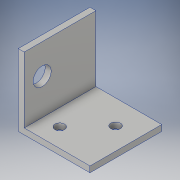
# Autodesk Inventor part: CLB_085_ClimberMountLBracket
Saved by Autodesk Inventor 2018.3 (Build 223284000, 284)
## iProperties
Created: 2020-02-22
Part Number: CLB_085_ClimberMountLBracket
Material: Aluminum 6061
Document SubType Name: Modeling
Designer: 22perngrac
Density: 2.7 g/cm^3
Appearance: Aluminum - Flat
Mass: 22.9264 g
Surface Area: 62.4575 cm^2
Volume: 8.49126 cm^3
Author: 22perngrac
Autodesk Inventor part; units mm, degrees
ref_plane "YZ Plane" through (0, 0, 0) normal (1, 0, 0) x (0, 1, 0)
ref_plane "XZ Plane" through (0, 0, 0) normal (0, 1, 0) x (-1, 0, 0)
ref_plane "XY Plane" through (0, 0, 0) normal (0, 0, 1) x (1, 0, 0)
sketch "Sketch1" plane through (0, 0, 0) normal (0, 0, 1) x (1, 0, 0)
  line L0 (0, 0) -> (0, 38.1)
  line L1 (0, 38.1) -> (3.175, 38.1)
  line L2 (3.175, 38.1) -> (3.175, 3.175)
  line L3 (3.175, 3.175) -> (38.1, 3.175)
  line L4 (38.1, 3.175) -> (38.1, 0)
  line L5 (38.1, 0) -> (0, 0)
  dimension "d0" = 38.1
  dimension "d1" = 3.175
  constraints: 12 end point, 7 perpendicular, 1 vertical
  measures "d0" distance of L4.end L0.start
  measures "d1" distance of L3.end L4.end
extrude "Extrusion1" add sketch "Sketch1" along normal blind 38.1
sketch "Sketch2" plane through (3.175, 3.175, 0) normal (1, 0, 0) x (0, 0, -1)
  line L0 (0, 34.925) -> (-38.1, 34.925) projected
  line L1 (-38.1, 0) -> (-38.1, 34.925) projected
  line L2 (0, 0) -> (-38.1, 0) projected
  point P0 (0, -3.175)
  point P1 (-28.575, 19.05)
  dimension "d5" = 9.525
  dimension "d24" = 19.05
  measures "d5" distance from line of L1 point (-28.575, 19.05)
  measures "d24" distance from line of point (-28.575, 19.05) L2
hole "Hole1" at (3.175, 22.225, 28.575) direction (-1, 0, 0) diameter 9.525 end through all
sketch "Sketch3" plane through (3.175, 3.175, 0) normal (0, 1, 0) x (1, 0, 0)
  line L0 (34.925, -38.1) -> (0, -38.1) projected
  line L1 (0, 0) -> (0, -38.1) projected
  line L2 (34.925, 0) -> (34.925, -38.1) projected
  point P0 (-3.175, 0)
  point P1 (8.9154, -28.1686)
  point P2 (23.3172, -12.8778)
  dimension "d13" = 9.9314
  dimension "d14" = 8.9154
  dimension "d15" = 25.2222
  dimension "d16" = 11.6078
  measures "d13" distance from line of L0 point (8.915, -28.169)
  measures "d14" distance from line of L1 point (8.915, -28.169)
  measures "d15" distance from line of L0 point (23.317, -12.878)
  measures "d16" distance from line of L2 point (23.317, -12.878)
hole "Hole2" at (12.0904, 3.175, 28.1686) at (26.4922, 3.175, 12.8778) direction (0, -1, 0) diameter 5.1054 end through all
body "Solid1"
